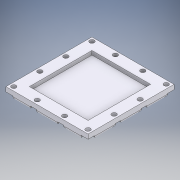
# Autodesk Inventor part: lid
Saved by Autodesk Inventor 2018 (Build 220112000, 112)
## iProperties
Created: 2019-05-28
Part Number: lid
Material: Generic
Document SubType Name: Modeling
Designer: ZEUSLAP
Density: 1 g/cm^3
Appearance: Default
Mass: 16.7192 g
Surface Area: 107.984 cm^2
Volume: 16.7192 cm^3
Author: ZEUSLAP
## iProperties of the stored document lid_3DPrint.ipt
Created: 2019-06-02
Part Number: lid_3DPrint
Material: Generic
Document SubType Name: Modeling
Designer: ZEUSLAP
Density: 1 g/cm^3
Appearance: Default
Author: ZEUSLAP
Autodesk Inventor part; units mm, degrees
ref_plane "YZ Plane" through (0, 0, 0) normal (1, 0, 0) x (0, 1, 0)
ref_plane "XZ Plane" through (0, 0, 0) normal (0, 1, 0) x (-1, 0, 0)
ref_plane "XY Plane" through (0, 0, 0) normal (0, 0, 1) x (1, 0, 0)
sketch "back_wall&m3_bolts" plane through (0, 0, 0) normal (0, 0, 1) x (1, 0, 0)
  circle A0 centre (-28.5, -10) radius 1.75
  line L0 (-36.4635, 0) -> (65.4635, 0) construction
  circle A1 centre (-28.5, -30) radius 1.75
  circle A2 centre (-10.5, -30) radius 1.75
  circle A3 centre (10.5, -30) radius 1.75
  circle A4 centre (28.5, -30) radius 1.75
  circle A5 centre (28.5, -10) radius 1.75
  circle A6 centre (28.5, 10) radius 1.75
  circle A7 centre (28.5, 30) radius 1.75
  circle A8 centre (10.5, 30) radius 1.75
  circle A9 centre (-10.5, 30) radius 1.75
  circle A10 centre (-28.5, 30) radius 1.75
  circle A11 centre (-28.5, 10) radius 1.75
  line L1 (0, 39.7442) -> (0, -45.329) construction
  line L2 (-31.5, -33) -> (31.5, -33)
  line L3 (31.5, -33) -> (31.5, 33)
  line L4 (31.5, 33) -> (-31.5, 33)
  line L5 (-31.5, 33) -> (-31.5, -33)
  line L6 (-26.4793, 26.5) -> (-30.5207, 26.5)
  line L7 (-30.5207, 26.5) -> (-32.5415, 30)
  line L8 (-32.5415, 30) -> (-30.5207, 33.5)
  line L9 (-30.5207, 33.5) -> (-26.4793, 33.5)
  line L10 (-26.4793, 33.5) -> (-24.4585, 30)
  line L11 (-24.4585, 30) -> (-26.4793, 26.5)
  line L12 (-8.4793, 26.5) -> (-12.5207, 26.5)
  line L13 (-12.5207, 26.5) -> (-14.5415, 30)
  line L14 (-14.5415, 30) -> (-12.5207, 33.5)
  line L15 (-12.5207, 33.5) -> (-8.4793, 33.5)
  line L16 (-8.4793, 33.5) -> (-6.4585, 30)
  line L17 (-6.4585, 30) -> (-8.4793, 26.5)
  line L18 (32.5415, 30) -> (30.5207, 26.5)
  line L19 (30.5207, 26.5) -> (26.4793, 26.5)
  line L20 (26.4793, 26.5) -> (24.4585, 30)
  line L21 (24.4585, 30) -> (26.4793, 33.5)
  line L22 (26.4793, 33.5) -> (30.5207, 33.5)
  line L23 (30.5207, 33.5) -> (32.5415, 30)
  line L24 (26.4793, 6.5) -> (24.4585, 10)
  line L25 (24.4585, 10) -> (26.4793, 13.5)
  line L26 (26.4793, 13.5) -> (30.5207, 13.5)
  line L27 (30.5207, 13.5) -> (32.5415, 10)
  line L28 (32.5415, 10) -> (30.5207, 6.5)
  line L29 (30.5207, 6.5) -> (26.4793, 6.5)
  line L30 (26.4793, -13.5) -> (24.4585, -10)
  line L31 (24.4585, -10) -> (26.4793, -6.5)
  line L32 (26.4793, -6.5) -> (30.5207, -6.5)
  line L33 (30.5207, -6.5) -> (32.5415, -10)
  line L34 (32.5415, -10) -> (30.5207, -13.5)
  line L35 (30.5207, -13.5) -> (26.4793, -13.5)
  line L36 (26.4793, -33.5) -> (24.4585, -30)
  line L37 (24.4585, -30) -> (26.4793, -26.5)
  line L38 (26.4793, -26.5) -> (30.5207, -26.5)
  line L39 (30.5207, -26.5) -> (32.5415, -30)
  line L40 (32.5415, -30) -> (30.5207, -33.5)
  line L41 (30.5207, -33.5) -> (26.4793, -33.5)
  line L42 (8.4793, -26.5) -> (12.5207, -26.5)
  line L43 (12.5207, -26.5) -> (14.5415, -30)
  line L44 (14.5415, -30) -> (12.5207, -33.5)
  line L45 (12.5207, -33.5) -> (8.4793, -33.5)
  line L46 (8.4793, -33.5) -> (6.4585, -30)
  line L47 (6.4585, -30) -> (8.4793, -26.5)
  line L48 (-8.4793, -26.5) -> (-6.4585, -30)
  line L49 (-6.4585, -30) -> (-8.4793, -33.5)
  line L50 (-8.4793, -33.5) -> (-12.5207, -33.5)
  line L51 (-12.5207, -33.5) -> (-14.5415, -30)
  line L52 (-14.5415, -30) -> (-12.5207, -26.5)
  line L53 (-12.5207, -26.5) -> (-8.4793, -26.5)
  line L54 (-26.4793, -26.5) -> (-24.4585, -30)
  line L55 (-24.4585, -30) -> (-26.4793, -33.5)
  line L56 (-26.4793, -33.5) -> (-30.5207, -33.5)
  line L57 (-30.5207, -33.5) -> (-32.5415, -30)
  line L58 (-32.5415, -30) -> (-30.5207, -26.5)
  line L59 (-30.5207, -26.5) -> (-26.4793, -26.5)
  line L60 (-26.4793, -13.5) -> (-30.5207, -13.5)
  line L61 (-30.5207, -13.5) -> (-32.5415, -10)
  line L62 (-32.5415, -10) -> (-30.5207, -6.5)
  line L63 (-30.5207, -6.5) -> (-26.4793, -6.5)
  line L64 (-26.4793, -6.5) -> (-24.4585, -10)
  line L65 (-24.4585, -10) -> (-26.4793, -13.5)
  line L66 (-26.4793, 6.5) -> (-30.5207, 6.5)
  line L67 (-30.5207, 6.5) -> (-32.5415, 10)
  line L68 (-32.5415, 10) -> (-30.5207, 13.5)
  line L69 (-30.5207, 13.5) -> (-26.4793, 13.5)
  line L70 (-26.4793, 13.5) -> (-24.4585, 10)
  line L71 (-24.4585, 10) -> (-26.4793, 6.5)
  line L72 (30.8094, 33) -> (31.5, 33)
  line L73 (31.5, 33) -> (31.5, 31.8038)
  line L74 (31.5, -31.8038) -> (31.5, -33)
  line L75 (31.5, -33) -> (30.8094, -33)
  line L76 (-31.5, -31.8038) -> (-31.5, -33)
  line L77 (-31.5, -33) -> (-30.8094, -33)
  line L78 (-30.8094, 33) -> (-31.5, 33)
  line L79 (-31.5, 31.8038) -> (-31.5, 33)
  circle A12 centre (10.5, 30) radius 3.25
  point P0 (0, 0)
  point P1 (14.5, 0)
  point P2 (0, 0)
  point P3 (0, 33)
  point P4 (31.5, 0)
  dimension "d0" = 3.5
  dimension "d1" = 10
  dimension "d3" = 20
  dimension "d5" = 63
  dimension "d6" = 66
  dimension "d11" = 3.5
  dimension "d12" = 10.5
  dimension "d16" = 3
  dimension "d17" = 3
  dimension "d18" = 18
  dimension "d19" = 20
  dimension "d26" = 6.5
  constraints: 160 end point, 18 point on line, 15 coincident, 13 centre point, 11 equal radius, 5 collinear, 4 horizontal, 4 vertical alignment, 3 midpoint, 3 parallel, 2 perpendicular, 2 symmetric about line, 1 horizontal alignment, 1 vertical, 155 other
  measures "d0" diameter of A0
  measures "d1" distance from line of L0 A0.centre
  measures "d3" distance of A1.centre A0.centre
  measures "d5" distance of L3.end L4.end
  measures "d6" distance of L2.end L3.end
  measures "d11" distance from line of L9 point (-28.5, 30)
  measures "d12" distance from line of L1 A9.centre
  measures "d16" distance from line of L4 A10.centre
  measures "d17" distance from line of L5 A10.centre
  measures "d18" distance of A9.centre A10.centre
  measures "d19" distance of A11.centre A10.centre
  measures "d26" diameter of A12
extrude "wall" add sketch "back_wall&m3_bolts" along normal blind 3 contours A0 | A1 | A2 | A3 | A4 | A5 | A6 | A7 | A8 | A9 | A10 | A11 | L5 L57 L2 | L57 L5 L58 L59 L54 L55 L2 | L55 L54 L59 L58 L5 L61 L60 L65 L64 L63 L62 L67 L66 L71 L70 L69 L68 L7 L6 L11 L10 L4 L14 L13 L12 L17 L16 A12 L21 L20 L19 L18 L3 L27 L26 L25 L24 L29 L28 L33 L32 L31 L30 L35 L34 L39 L38 L37 L36 L2 L44 L43 L42 L47 L46 L49 L48 L53 L52 L51 | L51 L52 L53 L48 L49 L2 | L5 L62 L63 L64 L65 L60 L61 | L46 L47 L42 L43 L44 L2 | L5 L68 L69 L70 L71 L66 L67 | L36 L37 L38 L39 L3 L40 L2 | L5 L8 L4 L10 L11 L6 L7 | L40 L3 L2 | L5 L4 L8 | L34 L35 L30 L31 L32 L33 L3 | L4 L16 L17 L12 L13 L14 | L28 L29 L24 L25 L26 L27 L3 | L4 A12 | L18 L19 L20 L21 L4 L23 L3 | L23 L4 L3 picked at (10.4297, 32.5791)
sketch "lipSketch" plane through (0, 0, 3) normal (0, 0, 1) x (1, 0, 0)
  line L0 (31.5, 33) -> (-31.5, 33) projected
  line L1 (-31.5, 33) -> (-31.5, -33) projected
  line L2 (-31.5, -33) -> (31.5, -33) projected
  line L3 (31.5, -33) -> (31.5, 33) projected
  line L4 (-22.5, 24) -> (22.5, 24)
  line L5 (22.5, 24) -> (22.5, -24)
  line L6 (22.5, -24) -> (-22.5, -24)
  line L7 (-22.5, -24) -> (-22.5, 24)
  point P0 (0, 0)
  dimension "d22" = 9
  constraints: 8 end point, 3 other
  measures "d22" distance between parallel lines of L0 L4
extrude "lip" add sketch "lipSketch" along normal blind 3
extrude "m3_bolt_holes" cut sketch "back_wall&m3_bolts" along normal through all contours A0 | A1 | A2 | A3 | A4 | A5 | A6 | A7 | A8 | A9 | A10 | A11
extrude "m3_nut_slots" cut sketch "back_wall&m3_bolts" along normal blind 2.5 contours L5 L57 L2 | L57 L5 L58 L59 L54 L55 L2 | L2 L55 L56 L57 | L57 L58 L5 | L51 L52 L53 L48 L49 L2 | L2 L49 L50 L51 | L61 L62 L5 | L5 L62 L63 L64 L65 L60 L61 | L46 L47 L42 L43 L44 L2 | L2 L44 L45 L46 | L67 L68 L5 | L5 L68 L69 L70 L71 L66 L67 | L36 L37 L38 L39 L3 L40 L2 | L2 L40 L41 L36 | L7 L8 L5 | L5 L8 L4 L10 L11 L6 L7 | L40 L3 L2 | L5 L4 L8 | L3 L39 L40 | L8 L9 L10 L4 | L34 L35 L30 L31 L32 L33 L3 | L3 L33 L34 | L14 L15 L16 L4 | L4 L16 L17 L12 L13 L14 | L28 L29 L24 L25 L26 L27 L3 | L3 L27 L28 | A12 L4 | L4 A12 | L18 L19 L20 L21 L4 L23 L3 | L3 L23 L18 | L21 L22 L23 L4 | L23 L4 L3
fillet "Fillet1" radius 2 12 edges at (31.5, -20, 0) (19.5, -33, 0) (0, -33, 0) (-19.5, -33, 0) (-31.5, -20, 0) (-31.5, 0, 0) (-31.5, 20, 0) (-19.5, 33, 0) (18.9703, 33, 0) (0.5297, 33, 0) (31.5, 20, 0) (31.5, 0, 0)
body "Solid1"
